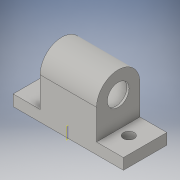
# Autodesk Inventor part: Part2
Saved by Autodesk Inventor 2016 (Build 200138000, 138)
## iProperties
Created: 2016-04-20
Part Number: Part2
Material: Generic
Document SubType Name: Modeling
Designer: Scott
Density: 1 g/cm^3
Appearance: Default
Author: Scott
Autodesk Inventor part; units mm, degrees
ref_plane "YZ Plane" through (0, 0, 0) normal (1, 0, 0) x (0, 1, 0)
ref_plane "XZ Plane" through (0, 0, 0) normal (0, 1, 0) x (-1, 0, 0)
ref_plane "XY Plane" through (0, 0, 0) normal (0, 0, 1) x (1, 0, 0)
sketch "Sketch1" plane through (0, 0, 0) normal (0, 1, 0) x (-1, 0, 0)
  line L0 (25.4, -10) -> (-25.4, -10)
  line L1 (-25.4, -10) -> (-25.4, 10)
  line L2 (-25.4, 10) -> (25.4, 10)
  line L3 (25.4, 10) -> (25.4, -10)
  line L4 (25.4, -10) -> (-25.4, 10) construction
  line L5 (-25.4, -10) -> (25.4, 10) construction
  circle A0 centre (-17.9, 0) radius 2.5
  circle A1 centre (17.9, 0) radius 2.5
  point P0 (0, 0)
  dimension "d0" = 50.8
  dimension "d1" = 20
  dimension "d2" = 5
  dimension "d3" = 5
  dimension "d4" = 7.5
  dimension "d5" = 7.5
  constraints: 12 end point, 2 centre point, 2 midpoint, 2 parallel, 1 horizontal, 1 perpendicular
  measures "d0" distance of L1.end L2.end
  measures "d1" distance of L0.end L1.end
  measures "d2" diameter of A0
  measures "d3" diameter of A1
  measures "d4" distance from line of L3 A1.centre
  measures "d5" distance from line of L1 A0.centre
extrude "Extrusion1" add sketch "Sketch1" along normal blind 5.08
ref_plane "Work Plane1" through (0, 0, -10) normal (-1, 0, 0) x (0, 0, 1)
sketch "Sketch2" plane through (0, 0, -10) normal (-1, 0, 0) x (0, 0, 1)
  line L0 (0, 0) -> (20, 0) projected
  line L1 (0, 0) -> (0, 5.08) projected
  line L2 (20, 5.08) -> (0, 5.08) projected
  line L3 (20, 0) -> (20, 5.08) projected
  line L4 (0, 5.08) -> (20, 5.08) projected
  line L5 (10, 0) -> (10, 2.54)
  line L6 (10, 5.08) -> (10, 11.43)
  line L7 (10, 11.43) -> (10, 18.93)
  circle A0 centre (10, 18.93) radius 7.5
  line L8 (20, 5.08) -> (20, 18.93)
  line L9 (0, 5.08) -> (0, 18.93)
  arc A1 (20, 18.93) -> (0, 18.93) centre (10, 18.93) ccw
  line L10 (20, 18.93) -> (20, 5.08)
  line L11 (20, 5.08) -> (0, 5.08)
  line L12 (0, 5.08) -> (0, 18.93)
  dimension "d10" = 2.54
  dimension "d11" = 6.35
  dimension "d12" = 7.5
  dimension "d13" = 15
  constraints: 16 end point, 5 vertical, 2 centre point, 2 coincident, 2 collinear, 2 point on circle, 1 midpoint, 1 point on line
  measures "d10" distance of L5.start L5.end
  measures "d11" distance of L6.start L6.end
  measures "d12" distance of L6.end L7.end
  measures "d13" diameter of A0
extrude "Extrusion2" add sketch "Sketch2" along normal mid plane 24 contours L9 A1 L8 L2
sketch "Sketch3" plane through (12, 0, -10) normal (1, 0, 0) x (0, 0, -1)
  circle A0 centre (-10, 18.93) radius 7.5 projected
  line L0 (0, 5.08) -> (-20, 5.08) projected
  line L1 (0, 5.08) -> (0, 18.93) projected
  arc A1 (0, 18.93) -> (-20, 18.93) centre (-10, 18.93) ccw projected
  line L2 (-20, 18.93) -> (-20, 5.08) projected
  circle A2 centre (-10, 18.93) radius 5
  point P0 (-10, 0)
  dimension "d16" = 10
  constraints: 1 centre point, 1 coincident
  measures "d16" diameter of A2
extrude "Extrusion3" add sketch "Sketch3" along normal blind 1 contours A0 | L0 L2 A1 L1
sketch "Sketch4" plane through (-12, 0, -10) normal (-1, 0, 0) x (0, 0, 1)
  circle A0 centre (10, 18.93) radius 7.5 projected
  line L0 (20, 5.08) -> (0, 5.08) projected
  line L1 (20, 5.08) -> (20, 18.93) projected
  arc A1 (20, 18.93) -> (0, 18.93) centre (10, 18.93) ccw projected
  line L2 (0, 18.93) -> (0, 5.08) projected
  point P0 (10, 0)
extrude "Extrusion4" add sketch "Sketch4" along normal blind 1
body "Solid1"
